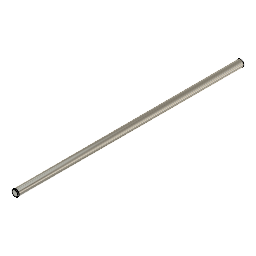
Linear_rail_Y_F01 (Autodesk Fusion 360 design; units mm, degrees)
Autodesk Fusion 360 part; units mm, degrees
cylinder "円柱プリミティブ1" add diameter 10 height 320 placed x (1, 0, 0) y (0, 0, -1) z (0, 1, 0) at (0, 0, 0)
chamfer "面取り1" distance 1 angle 45 2 edges at (-4.6616, 320, 1.8081) (-4.6616, 0, -1.8081)
